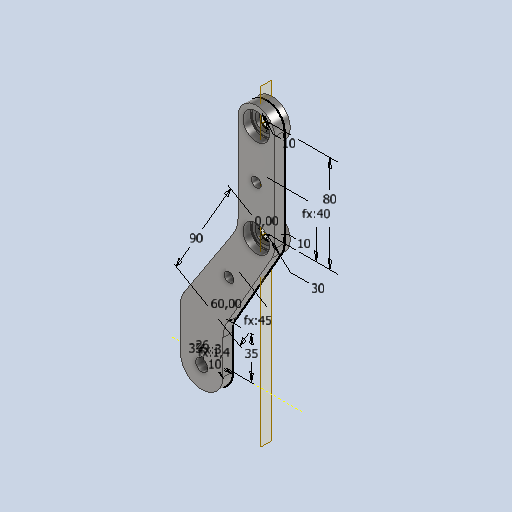
# Autodesk Inventor part: ParallelSystem_ProximalPart_Driven_v2
Saved by Autodesk Inventor 2022 (Build 260153000, 153)
## iProperties
Created: 2022-07-18
Part Number: ParallelSystem_ProximalPart_Driven_v2
Material: Edelstahl
Document SubType Name: Modeling
Designer: alexw
Density: 8 g/cm^3
Appearance: Halbpoliert
Mass: 237.14 g
Surface Area: 170.01 cm^2
Volume: 29.6426 cm^3
d0: 10,000 mm
d1: 26,000 mm
d4: 35,000 mm
d7: 5,000 mm
d8: 0,00 grd
d9: 6,000 mm
d10: 0,00 grd
d11: 25,000 mm
d23: 8,000 mm
d36: 0,00 grd
d37: 30,000 mm
d38: 60,00 grd
d39: 35,000 mm
d40: 90,000 mm
d41: 80,000 mm
d42: 45,000 mm
d43: 10,000 mm
d44: 10,000 mm
d45: 40,000 mm
Passfeder_width: 3,000 mm
Nabennuttiefe: 1,400 mm
d51: 3,000 mm
d52: 1,400 mm
ParallelLink_BearingStep_Height: 5,000 mm
ParallelLink_Lever_Thickness: 8,000 mm
Author: alexw
Autodesk Inventor part; units mm, degrees
ref_plane "YZ Plane" through (0, 0, 0) normal (1, 0, 0) x (0, 1, 0)
ref_plane "XZ Plane" through (0, 0, 0) normal (0, 1, 0) x (-1, 0, 0)
ref_plane "XY Plane" through (0, 0, 0) normal (0, 0, 1) x (1, 0, 0)
sketch "Skizze1" plane through (0, 0, 0) normal (0, 0, 1) x (1, 0, 0)
  arc A0 (-1.5, 4.7697) -> (1.5, 4.7697) centre (0, 0) ccw
  circle A1 centre (0, 0) radius 13
  line L0 (-33.9343, 0) -> (76.2277, 0) construction
  circle A2 centre (0, 0) radius 17.5
  circle A3 centre (45, 112.9423) radius 15
  line L1 (60, 112.9423) -> (60, 192.9423)
  line L2 (30, 112.9423) -> (30, 192.9423)
  line L3 (45, 112.9423) -> (45, 207.9423) construction
  line L4 (45, 112.9423) -> (45, 127.9423) construction
  line L5 (30, 112.9423) -> (60, 112.9423) construction
  line L6 (-17.5, 0) -> (-17.5, 35)
  line L7 (17.5, 0) -> (17.5, 35)
  line L8 (-17.5, 35) -> (17.5, 35) construction
  circle A4 centre (0, 35) radius 17.5 construction
  line L9 (-14.6522, 44.5688) -> (30, 112.9423)
  arc A5 (-14.6522, 44.5688) -> (-17.5, 35) centre (0, 35) ccw
  line L10 (17.5, 35) -> (58.0047, 105.4671)
  arc A6 (58.0047, 105.4671) -> (60, 112.9423) centre (45, 112.9423) ccw
  line L11 (0, 35) -> (45, 112.9423) construction
  circle A7 centre (45, 192.9423) radius 15
  circle A8 centre (45, 192.9423) radius 5
  circle A9 centre (45, 112.9423) radius 5
  line L12 (-1.5, 6.4) -> (1.5, 6.4)
  line L13 (1.5, 6.4) -> (1.5, 4.7697)
  line L14 (-1.5, 4.7697) -> (-1.5, 6.4)
  line L15 (0, 0) -> (0, 5) construction
  line L16 (0, 5) -> (1.5, 5) construction
  point P0 (22.5, 73.9711)
  point P1 (45, 152.9423)
  point P2 (-13, 0)
  point P3 (13, 0)
  point P4 (0, 6.4)
  dimension "d0" = 10
  dimension "d1" = 26
  dimension "d4" = 35
  dimension "d36" = 0
  dimension "d37" = 30
  dimension "d38" = 60
  dimension "d39" = 35
  dimension "d40" = 90
  dimension "d41" = 80
  dimension "d42" = 45
  dimension "d43" = 10
  dimension "d44" = 10
  dimension "d45" = 40
  dimension "d51" = 3
  dimension "d52" = 1.4
  constraints: 32 end point, 17 point on circle, 13 tangent, 10 centre point, 8 point on line, 6 coincident, 5 perpendicular, 4 midpoint, 2 equal radius, 2 horizontal, 2 parallel, 2 vertical
  measures "d0" diameter of A0
  measures "d1" diameter of A1
  measures "d4" diameter of A2
  measures "d36" distance between parallel lines of L3 L4
  measures "d37" diameter of A3
  measures "d38" angle of L8 L11
  measures "d39" distance of A4.centre point (0, 0)
  measures "d40" distance of point (45, 112.942) A4.centre
  measures "d41" distance of A7.centre point (45, 112.942)
  measures "d42" distance of point (22.5, 73.971) A4.centre
  measures "d43" diameter of A8
  measures "d44" diameter of A9
  measures "d45" distance of point (45, 152.942) point (45, 112.942)
  measures "d51" distance of L12.start L12.end
  measures "d52" distance between parallel lines of L12 L16
extrude "Extrusion1" add sketch "Skizze1" against normal blind 5 contours A1 | A3 | A7
extrude "Extrusion2" add sketch "Skizze1" along normal blind 8 contours A1 | A2 | A2 L6 A5 L9 A3 L10 L7 | A3 | L2 A7 L1 A3 | A7
fillet "Rundung1" radius 25 2 edges at (30, 112.9423, 4) (17.5, 35, 4)
hole "Bohrung2" at (45, 152.9423, 0) at (22.5, 73.9711, 0) direction (0, 0, 1) diameter 8 end through all
ref_plane "Arbeitsebene1" through (45, 112.9423, 0) normal (1, 0, 0) x (0, 0, -1)
sketch "Skizze3" plane through (45, 112.9423, 0) normal (1, 0, 0) x (0, 0, -1)
  line L0 (-10.6, 0) -> (7.6, 0) construction
  line L1 (-10.6, 80) -> (7.6, 80) construction
  line L2 (-8, 91) -> (-2, 91)
  line L3 (-2, 91) -> (-2, 90)
  line L4 (-2, 90) -> (-1.5, 90)
  line L5 (-1.5, 90) -> (-1.5, 87.5)
  line L6 (-1.5, 87.5) -> (2, 87.5)
  line L7 (-8, 75) -> (-8, 85) construction
  line L8 (5, 85) -> (-8, 85) construction
  line L9 (5, 75) -> (-8, 75) construction
  line L10 (5, 85) -> (5, 75) construction
  line L11 (0, 0) -> (0, 80) construction
  line L12 (2, 87.5) -> (2, 92)
  line L13 (2, 92) -> (5, 92)
  line L14 (-8, 91) -> (-8, 85)
  line L15 (5, 92) -> (5, 85)
  line L16 (-8, 85) -> (5, 85)
  point P0 (0, -112.9423)
  dimension "d53" = 6
  dimension "d54" = 22
  dimension "d55" = 20
  dimension "d56" = 15
  dimension "d57" = 24
  dimension "d58" = 3
  dimension "d59" = 0.5
  constraints: 20 end point, 7 perpendicular, 2 horizontal, 2 point on line, 1 vertical
  measures "d53" distance of L2.start L2.end
  measures "d54" diameter of L2 L1
  measures "d55" diameter of L4 L1
  measures "d56" diameter of L6 L1
  measures "d57" diameter of L13 L1
  measures "d58" distance from line of L13.end L12
  measures "d59" distance between parallel lines of L3 L5
revolve "Umdrehung1" cut sketch "Skizze3" angle 360 about axis through (45, 192.9423, 0) along (0, 0, -1)
pattern_linear "Rechteckige Anordnung1" count 2 spacing 80 along (0, -1, 0) of "Umdrehung1"
